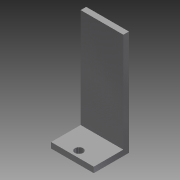
# Autodesk Inventor part: L Bracket
Saved by Autodesk Inventor 2013 (Build 170138000, 138)
## iProperties
Created: 2014-07-18
Part Number: L Bracket
Material: Steel, Galvanized
Document SubType Name: Modeling
Designer: Kyle
Density: 1 g/cm^3
Author: Kyle
Autodesk Inventor part; units mm, degrees
ref_plane "YZ Plane" through (0, 0, 0) normal (1, 0, 0) x (0, 1, 0)
ref_plane "XZ Plane" through (0, 0, 0) normal (0, 1, 0) x (-1, 0, 0)
ref_plane "XY Plane" through (0, 0, 0) normal (0, 0, 1) x (1, 0, 0)
sketch "Sketch1" plane through (0, 0, 0) normal (0, 0, 1) x (1, 0, 0)
  line L0 (0, 0) -> (16.51, 0)
  line L1 (16.51, 0) -> (16.51, 40.64)
  line L2 (16.51, 40.64) -> (0, 40.64)
  line L3 (0, 40.64) -> (0, 0)
  dimension "d0" = 40.64
  dimension "d1" = 16.51
  constraints: 8 end point, 2 parallel, 1 horizontal, 1 perpendicular
  measures "d0" distance of L2.end L0.start
  measures "d1" distance of L0.start L0.end
extrude "Extrusion1" add sketch "Sketch1" along normal blind 2.159
sketch "Sketch2" plane through (0, 0, 2.159) normal (0, 0, 1) x (1, 0, 0)
  line L0 (0, 0) -> (16.51, 0) projected
  line L1 (16.51, 0) -> (16.51, 40.64) projected
  line L2 (0, 0) -> (16.51, 0)
  line L3 (16.51, 0) -> (16.51, 2.159)
  line L4 (16.51, 2.159) -> (0, 2.159)
  line L5 (0, 2.159) -> (0, 0)
  dimension "d4" = 2.159
  constraints: 8 end point, 2 parallel, 1 horizontal, 1 perpendicular, 1 point on line
  measures "d4" distance between parallel lines of L4 L2
extrude "Extrusion2" add sketch "Sketch2" along normal blind 11.43
sketch "Sketch3" plane through (0, 2.159, 2.159) normal (0, 1, 0) x (1, 0, 0)
  circle A0 centre (8.255, -8.89) radius 1.5875
  line L0 (16.51, -11.43) -> (0, -11.43) projected
  point P0 (0, 2.159)
  dimension "d8" = 3.175
  dimension "d12" = 2.54
  constraints: 1 centre point
  measures "d8" diameter of A0
  measures "d12" distance from line of L0 A0.centre
extrude "Extrusion3" cut sketch "Sketch3" against normal blind 11.43
body "Solid1"
